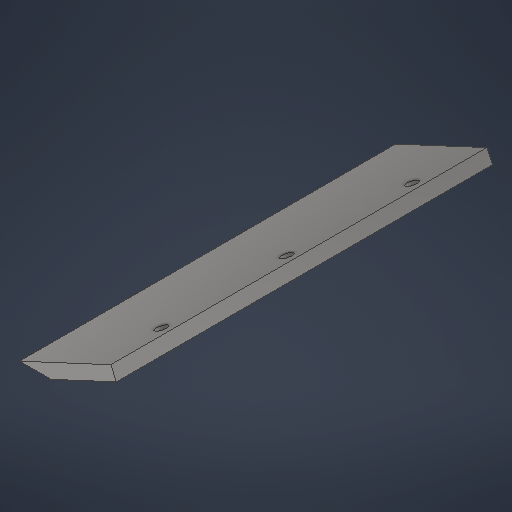
# Autodesk Inventor part: lowerRamp
Saved by Autodesk Inventor 2025 (Build 290162000, 162)
## iProperties
Created: 2025-03-14
Part Number: lowerRamp
Material: Ocel, uhlík
Document SubType Name: Modeling
Designer: Simak
Density: 7.85 g/cm^3
Appearance: Pololeštěná
Author: Simak
Autodesk Inventor part; units mm, degrees
ref_plane "YZ Plane" through (0, 0, 0) normal (1, 0, 0) x (0, 1, 0)
ref_plane "XZ Plane" through (0, 0, 0) normal (0, 1, 0) x (-1, 0, 0)
ref_plane "XY Plane" through (0, 0, 0) normal (0, 0, 1) x (1, 0, 0)
sketch "Náčrt1" plane through (0, 0, 0) normal (0, 0, 1) x (1, 0, 0)
  line L0 (0, 0) -> (11.831, 0)
  line L1 (11.831, 0) -> (26.7952, 6.9779)
  line L2 (26.7952, 6.9779) -> (24.6821, 11.5094)
  line L3 (24.6821, 11.5094) -> (0, 0)
  line L4 (0, 0) -> (26.7952, 0) construction
  line L5 (18.5187, 6.9803) -> (25.316, 10.15) construction
  line L6 (25.316, 10.15) -> (24.2277, 7.1599) construction
  line L7 (24.2277, 7.1599) -> (26.6578, 1.9486) construction
  line L8 (26.6578, 1.9486) -> (23.9388, 0.6808) construction
  line L9 (23.9388, 0.6808) -> (21.5088, 5.892) construction
  line L10 (21.5088, 5.892) -> (18.5187, 6.9803) construction
  line L11 (23.7275, 1.1339) -> (22.3681, 0.5) construction
  line L12 (26.4465, 2.4018) -> (27.8059, 3.0357) construction
  line L13 (22.3681, 0.5) -> (21.5228, 2.3126) construction
  line L14 (21.5228, 2.3126) -> (26.9607, 4.8483) construction
  line L15 (26.9607, 4.8483) -> (27.8059, 3.0357) construction
  line L16 (50, 0) -> (58.2817, 0)
  line L17 (58.2817, 0) -> (75.5016, 8.0297)
  line L18 (75.5016, 8.0297) -> (74.0224, 11.2018)
  line L19 (74.0224, 11.2018) -> (50, 0)
  line L20 (50, 0) -> (75.5016, 0) construction
  line L21 (69.7022, 8.6356) -> (72.1322, 3.4243) construction
  line L22 (72.1322, 3.4243) -> (71.0439, 0.4342) construction
  line L23 (71.0439, 0.4342) -> (77.8412, 3.6039) construction
  line L24 (77.8412, 3.6039) -> (74.8511, 4.6922) construction
  line L25 (74.8511, 4.6922) -> (72.4211, 9.9034) construction
  line L26 (72.4211, 9.9034) -> (69.7022, 8.6356) construction
  line L27 (21.9174, 8.5652) -> (21.2834, 9.9246) construction
  line L28 (71.0616, 9.2695) -> (70.8503, 9.7227) construction
  dimension "d8" = 5
  dimension "d9" = 25
  dimension "d11" = 8
  dimension "d12" = 3
  dimension "d13" = 45
  dimension "d14" = 7.5
  dimension "d16" = 0
  dimension "d17" = 6
  dimension "d18" = 0.5
  dimension "d19" = 0.5
  dimension "d20" = 2
  dimension "d21" = 27.2337
  dimension "d22" = 3.5
  dimension "d23" = 25
  dimension "d34" = 26.5058
  dimension "d35" = 50
  dimension "d36" = 45
  dimension "d37" = 3
  dimension "d38" = 7.5
  dimension "d39" = 8
  dimension "d42" = 2
  dimension "d44" = 2
  dimension "d59" = 5
  dimension "d63" = 0.5
  dimension "d64" = 19
  dimension "d65" = 0.4342
  constraints: 58 end point, 13 perpendicular, 6 equal length, 6 point on line, 5 parallel, 2 coincident, 2 horizontal, 2 midpoint, 2 vertical alignment, 1 collinear, 1 horizontal alignment
  measures "d8" distance of L1.end L2.end
  measures "d9" angle of L0 L3
  measures "d11" distance between parallel lines of L8 L5
  measures "d12" distance of L7.end L8.end
  measures "d13" angle of L5 L6
  measures "d14" distance of L5.start L5.end
  measures "d16" distance from line of L2 L5.end
  measures "d17" distance of L12.end L11.end
  measures "d18" distance between parallel lines of L8 L12
  measures "d19" distance from line of L4 L11.end
  measures "d20" distance of L14.end L12.end
  measures "d21" distance of L2.end L0.start
  measures "d22" distance of L18.start L18.end
  measures "d23" angle of L16 L19
  measures "d34" distance of L18.end L16.start
  measures "d35" distance of point (0, 0) L16.start
  measures "d36" angle of L23 L24
  measures "d37" distance between parallel lines of L21 L25
  measures "d38" distance of L22.end L23.end
  measures "d39" distance between parallel lines of L26 L23
  measures "d42" distance between parallel lines of L18 L25
  measures "d44" distance between parallel lines of L1 L14
  measures "d59" distance between parallel lines of L17 L23
  measures "d63" distance between parallel lines of L19 L26
  measures "d64" distance of L16.end L18.start
  measures "d65" distance from line of L20 L22.end
extrude "Vysunutí1" add sketch "Náčrt1" along normal mid plane 99 contours L19 L18 L17 L16
sketch "Náčrt3" plane through (50, 0, 49.5) normal (-0.4226, 0.9063, 0) x (0.9063, 0.4226, 0)
  line L0 (23.0058, 49.5) -> (23.0058, 82.5) construction
  line L1 (23.0058, 82.5) -> (23.0058, 115.5) construction
  line L2 (0, 99) -> (26.5058, 99) projected
  line L3 (23.0058, 49.5) -> (23.0058, 16.5) construction
  point P0 (-45.3154, 49.5)
  point P1 (23.0058, 99)
  constraints: 6 end point, 2 coincident, 2 collinear, 2 point on line, 2 vertical, 1 midpoint
hole "Díra2" at (70.8503, 9.7227, 0) at (70.8503, 9.7227, -33) at (70.8503, 9.7227, 33) direction (0.4226, -0.9063, 0) diameter 3 end through all
thread "Závit1" size "M3x0.5" class "6H" standard "ANSI Metric M Profile" full length
thread "Závit2" size "M3x0.5" class "6H" standard "ANSI Metric M Profile" full length
thread "Závit3" size "M3x0.5" class "6H" standard "ANSI Metric M Profile" full length
